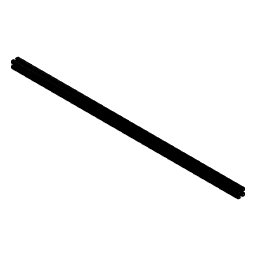
MakerBeam Profile 10x10x350 (Autodesk Fusion 360 design; units mm, degrees)
Autodesk Fusion 360 part; units mm, degrees
note: some values were not read from the file. Set by a fixed rule: which face or edge a step refers to.
sketch "Skizze1" plane through (0, 0, 0) normal (1, 0, 0) x (0, 0, -1)
  circle A0 centre (0, 0) radius 1.25
  line L0 (5, 5) -> (-5, -5) construction
  line L1 (-5, 5) -> (5, -5) construction
  line L2 (1, 2) -> (-1, 2)
  line L3 (-2, 1) -> (-2, -1)
  line L4 (-1, -2) -> (1, -2)
  line L5 (2, -1) -> (2, 1)
  line L6 (2, 2) -> (-2, -2) construction
  line L7 (-2, 2) -> (2, -2) construction
  line L8 (4, 4) -> (-4, -4) construction
  line L9 (-4, 4) -> (4, -4) construction
  line L10 (4.85, 1.5) -> (4.15, 1.5)
  line L11 (4.85, -1.5) -> (4.15, -1.5)
  line L12 (5, -4.95) -> (5, -1.65)
  line L13 (5, 1.65) -> (5, 4.95)
  line L14 (4, -3.0724) -> (4, -1.65)
  line L15 (4, 1.65) -> (4, 3.0724)
  line L16 (2, 1) -> (3.7329, 3.1661)
  line L17 (-20, 0) -> (18, 0) construction
  line L18 (0, 20) -> (0, -18) construction
  line L19 (2, -1) -> (3.7329, -3.1661)
  line L20 (-2, 1) -> (-3.7329, 3.1661)
  line L21 (-4.85, 1.5) -> (-4.15, 1.5)
  line L22 (-4.85, -1.5) -> (-4.15, -1.5)
  line L23 (-2, -1) -> (-3.7329, -3.1661)
  line L24 (-4, 3.0724) -> (-4, 1.65)
  line L25 (-4, -1.65) -> (-4, -3.0724)
  line L26 (-5, 4.95) -> (-5, 1.65)
  line L27 (-5, -1.65) -> (-5, -4.95)
  line L28 (-1, 2) -> (-3.1661, 3.7329)
  line L29 (-1.5, 4.85) -> (-1.5, 4.15)
  line L30 (1.5, 4.85) -> (1.5, 4.15)
  line L31 (1, 2) -> (3.1661, 3.7329)
  line L32 (3.0724, 4) -> (1.65, 4)
  line L33 (-1.65, 4) -> (-3.0724, 4)
  line L34 (4.95, 5) -> (1.65, 5)
  line L35 (-1.65, 5) -> (-4.95, 5)
  line L36 (-1, -2) -> (-3.1661, -3.7329)
  line L37 (-1.5, -4.85) -> (-1.5, -4.15)
  line L38 (1.5, -4.85) -> (1.5, -4.15)
  line L39 (1, -2) -> (3.1661, -3.7329)
  line L40 (-3.0724, -4) -> (-1.65, -4)
  line L41 (1.65, -4) -> (3.0724, -4)
  line L42 (-4.95, -5) -> (-1.65, -5)
  line L43 (1.65, -5) -> (4.95, -5)
  arc A1 (4.85, 1.5) -> (5, 1.65) centre (4.85, 1.65) ccw
  arc A2 (4, 1.65) -> (4.15, 1.5) centre (4.15, 1.65) ccw
  arc A3 (4, 3.0724) -> (3.7329, 3.1661) centre (3.85, 3.0724) ccw
  arc A4 (3.7329, -3.1661) -> (4, -3.0724) centre (3.85, -3.0724) ccw
  arc A5 (3.1661, 3.7329) -> (3.0724, 4) centre (3.0724, 3.85) ccw
  arc A6 (3.0724, -4) -> (3.1661, -3.7329) centre (3.0724, -3.85) ccw
  arc A7 (4.15, -1.5) -> (4, -1.65) centre (4.15, -1.65) ccw
  arc A8 (5, -1.65) -> (4.85, -1.5) centre (4.85, -1.65) ccw
  arc A9 (1.65, -4) -> (1.5, -4.15) centre (1.65, -4.15) ccw
  arc A10 (1.5, -4.85) -> (1.65, -5) centre (1.65, -4.85) ccw
  arc A11 (1.65, 5) -> (1.5, 4.85) centre (1.65, 4.85) ccw
  arc A12 (1.5, 4.15) -> (1.65, 4) centre (1.65, 4.15) ccw
  arc A13 (-1.5, 4.85) -> (-1.65, 5) centre (-1.65, 4.85) ccw
  arc A14 (-1.65, 4) -> (-1.5, 4.15) centre (-1.65, 4.15) ccw
  arc A15 (-3.0724, 4) -> (-3.1661, 3.7329) centre (-3.0724, 3.85) ccw
  arc A16 (-3.7329, 3.1661) -> (-4, 3.0724) centre (-3.85, 3.0724) ccw
  arc A17 (-5, 1.65) -> (-4.85, 1.5) centre (-4.85, 1.65) ccw
  arc A18 (-4.15, 1.5) -> (-4, 1.65) centre (-4.15, 1.65) ccw
  arc A19 (-4.85, -1.5) -> (-5, -1.65) centre (-4.85, -1.65) ccw
  arc A20 (-4, -1.65) -> (-4.15, -1.5) centre (-4.15, -1.65) ccw
  arc A21 (-4, -3.0724) -> (-3.7329, -3.1661) centre (-3.85, -3.0724) ccw
  arc A22 (-4.95, 5) -> (-5, 4.95) centre (-4.95, 4.95) ccw
  arc A23 (5, 4.95) -> (4.95, 5) centre (4.95, 4.95) ccw
  arc A24 (4.95, -5) -> (5, -4.95) centre (4.95, -4.95) ccw
  arc A25 (-5, -4.95) -> (-4.95, -5) centre (-4.95, -4.95) ccw
  arc A26 (-3.1661, -3.7329) -> (-3.0724, -4) centre (-3.0724, -3.85) ccw
  arc A27 (-1.5, -4.15) -> (-1.65, -4) centre (-1.65, -4.15) ccw
  arc A28 (-1.65, -5) -> (-1.5, -4.85) centre (-1.65, -4.85) ccw
  point P0 (5, 5)
  point P1 (5, 1.5)
  point P2 (5, 1.5)
  point P3 (5, -1.5)
  point P4 (4, 1.5)
  point P5 (2, 0)
  point P6 (4, 3.5)
  point P7 (4, -3.5)
  point P8 (0, 2)
  dimension "d1" = 2.5
  dimension "d2" = 10
  dimension "d5" = 4
  dimension "d6" = 8
  dimension "d8" = 3.5
  dimension "d9" = 3
  dimension "d11" = 1
  dimension "d12" = 2
  dimension "d13" = 2
  dimension "d14" = 1
  dimension "d15" = 0.15
  dimension "d16" = 0.15
  dimension "d17" = 0.15
  dimension "d18" = 0.15
  dimension "d19" = 0.15
  dimension "d20" = 0.15
  dimension "d21" = 0.15
  dimension "d22" = 0.15
  dimension "d23" = 0.15
  dimension "d24" = 0.15
  dimension "d25" = 0.15
  dimension "d26" = 0.15
  dimension "d27" = 0.15
  dimension "d28" = 0.15
  dimension "d29" = 0.15
  dimension "d30" = 0.15
  dimension "d31" = 0.15
  dimension "d32" = 0.15
  dimension "d33" = 0.15
  dimension "d34" = 0.15
  dimension "d35" = 0.15
  dimension "d36" = 0.05
  dimension "d37" = 0.05
  dimension "d38" = 0.05
  dimension "d39" = 0.05
  dimension "d40" = 0.15
  dimension "d41" = 0.15
  dimension "d42" = 0.15
  constraint coincident A0.centre origin
  constraint perpendicular L26 L34
  constraint parallel L34 L42
  constraint parallel L12 L26
  constraint horizontal L34
  constraint coincident L0 A0.centre
  constraint coincident L1 A0.centre
  constraint perpendicular L2 L3
  constraint parallel L2 L4
  constraint parallel L3 L5
  constraint horizontal L2
  constraint coincident L6 A0.centre
  constraint coincident L7 A0.centre
  constraint perpendicular L24 L32
  constraint parallel L32 L40
  constraint parallel L14 L24
  constraint horizontal L32
  constraint coincident L8 A0.centre
  constraint coincident L9 A0.centre
  constraint coincident P0 L0.start
  constraint coincident P2 L12
  constraint coincident P2 P1
  constraint coincident P4 L14
  constraint perpendicular L10 L14
  constraint perpendicular L11 L14
  constraint collinear L12 L13
  constraint collinear L14 L15
  constraint coincident L15 P6
  constraint coincident L5.end L16.start
  constraint horizontal L17
  constraint vertical L18
  constraint coincident L5 P5
  constraint symmetric P6 L17 P7
  constraint symmetric L5.end L17 L5.start
  constraint symmetric L5.end L18 L3.start
  constraint symmetric L18 L5.start L3.end
  constraint collinear L24 L25
  constraint collinear L26 L27
  constraint collinear L32 L33
  constraint collinear L34 L35
  constraint coincident L2 P8
  constraint symmetric L17 L2.start L4.end
  constraint symmetric L17 L2.end L4.start
  constraint collinear L40 L41
  constraint collinear L42 L43
  constraint tangent L13 A1
  constraint tangent L10 A1
  constraint coincident P4 L10
  constraint tangent L10 A2
  constraint tangent L15 A2
  constraint tangent L16 A3
  constraint tangent L15 A3
  constraint tangent L19 A4
  constraint tangent L14 A4
  constraint coincident L8.start L32
  constraint tangent L32 A5
  constraint tangent L31 A5
  constraint coincident L9.end L41
  constraint tangent L39 A6
  constraint tangent L41 A6
  constraint tangent L14 A7
  constraint tangent L11 A7
  constraint coincident P3 L12
  constraint tangent L11 A8
  constraint tangent L12 A8
  constraint tangent L41 A9
  constraint tangent L38 A9
  constraint tangent L38 A10
  constraint tangent L43 A10
  constraint tangent L34 A11
  constraint tangent L30 A11
  constraint tangent L30 A12
  constraint tangent L32 A12
  constraint tangent L35 A13
  constraint tangent L29 A13
  constraint tangent L29 A14
  constraint tangent L33 A14
  constraint coincident L9.start L33
  constraint tangent L33 A15
  constraint tangent L28 A15
  constraint coincident L9.start L24
  constraint tangent L20 A16
  constraint tangent L24 A16
  constraint tangent L26 A17
  constraint tangent L21 A17
  constraint tangent L24 A18
  constraint tangent L21 A18
  constraint tangent L27 A19
  constraint tangent L22 A19
  constraint tangent L22 A20
  constraint tangent L25 A20
  constraint coincident L8.end L25
  constraint tangent L25 A21
  constraint tangent L23 A21
  constraint coincident L1.start L26
  constraint coincident L1.start L35
  constraint tangent L26 A22
  constraint tangent L35 A22
  constraint coincident P0 L34
  constraint coincident P0 L13
  constraint tangent L34 A23
  constraint tangent L13 A23
  constraint coincident L1.end L12
  constraint coincident L1.end L43
  constraint tangent L12 A24
  constraint tangent L43 A24
  constraint coincident L0.end L27
  constraint coincident L0.end L42
  constraint tangent L27 A25
  constraint tangent L42 A25
  constraint coincident L8.end L40
  constraint tangent L36 A26
  constraint tangent L40 A26
  constraint tangent L40 A27
  constraint tangent L37 A27
  constraint tangent L37 A28
  constraint tangent L42 A28
  measures "d1" diameter of A0
  measures "d2" distance of L1.start L0.end
  measures "d5" distance of L7.start L6.end
  measures "d6" distance of L9.start L8.end
  measures "d8" distance of P0 P2
  measures "d9" distance of P2 P3
  measures "d11" distance of P5 L5.end
  measures "d12" distance of L5.end L5.start
  measures "d13" distance of P4 P6
  measures "d14" distance of P8 L2.end
  measures "d15" radius of A1
  measures "d16" radius of A2
  measures "d17" radius of A3
  measures "d18" radius of A4
  measures "d19" radius of A5
  measures "d20" radius of A6
  measures "d21" radius of A7
  measures "d22" radius of A8
  measures "d23" radius of A9
  measures "d24" radius of A10
  measures "d25" radius of A11
  measures "d26" radius of A12
  measures "d27" radius of A13
  measures "d28" radius of A14
  measures "d29" radius of A15
  measures "d30" radius of A16
  measures "d31" radius of A17
  measures "d32" radius of A18
  measures "d33" radius of A19
  measures "d34" radius of A20
  measures "d35" radius of A21
  measures "d36" radius of A22
  measures "d37" radius of A23
  measures "d38" radius of A24
  measures "d39" radius of A25
  measures "d40" radius of A26
  measures "d41" radius of A27
  measures "d42" radius of A28
extrude "Extrusion1" add sketch "Skizze1" along normal blind 350
thread "Gewinde1" "ISO Metric profile 3.0 M3x0.5 6H" major diameter 3.086 minor diameter 2.529 pitch 0.5 angle 60 modelled right hand crest width 0.1368 on face at (233.3333, -1.231, 0.2171) from (345, 0, 0) to (350, 0, 0) crest through (0.125, 0, -1.2645)
thread "Gewinde2" "ISO Metric profile 3.0 M3x0.5 6H" major diameter 3.086 minor diameter 2.529 pitch 0.5 angle 60 modelled right hand crest width 0.1368 on face at (230.0161, -1.0812, 0.6557) from (0, 0, 0) to (5, 0, 0) crest through (0.125, 0, -1.2645)
named bodies: "MakerBeam Profile 10x10x350"
